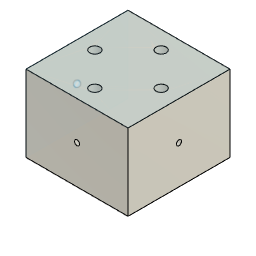
Suètone-drawing-object-02 (Autodesk Fusion 360 design; units mm, degrees)
Autodesk Fusion 360 part; units mm, degrees
sketch "Esquisse1" plane through (0, 0, 0) normal (0, 0, 1) x (1, 0, 0)
  line L0 (40, 40) -> (-40, 40)
  line L1 (-40, 40) -> (-40, -40)
  line L2 (-40, -40) -> (40, -40)
  line L3 (40, -40) -> (40, 40)
  line L4 (40, 40) -> (-40, -40) construction
  line L5 (-40, 40) -> (40, -40) construction
  dimension "d1" = 80
  dimension "d2" = 80
  constraint horizontal L0
  constraint perpendicular L0 L1
  constraint parallel L0 L2
  constraint parallel L1 L3
  constraint coincident L4 origin
  constraint coincident L5 origin
  measures "d1" distance of L1.end L2.end
  measures "d2" distance of L0.end L1.end
extrude "Extrusion1" add sketch "Esquisse1" along normal blind 80 makes body 1
sketch "Esquisse2" plane through (0, 0, 80) normal (0, 0, 1) x (-1, 0, 0)
  line L0 (-40, 40) -> (-40, -40)
  line L1 (-40, -40) -> (40, -40)
  line L2 (40, -40) -> (40, 40)
  line L3 (40, 40) -> (-40, 40)
  circle A0 centre (0, -26) radius 4
  circle A1 centre (26, 0) radius 4
  circle A2 centre (0, 26) radius 4
  circle A3 centre (-26, 0) radius 4
  dimension "d7" = 8
  dimension "d9" = 360
  measures "d7" diameter of A0
extrude "Extrusion2" cut sketch "Esquisse2" against normal blind 115 contours A0 | A1 | A2 | A3 bodies 1
sketch "Esquisse3" plane through (0, -40, 0) normal (0, -1, 0) x (1, 0, 0)
  line L0 (-40, 0) -> (40, 0)
  line L1 (40, 0) -> (40, 80)
  line L2 (40, 80) -> (-40, 80)
  line L3 (-40, 80) -> (-40, 0)
  line L4 (-40, 20) -> (40, 20)
  line L5 (40, 0, -80) -> (40, 80, -80)
  line L6 (40, 20, 0) -> (40, 20, -80)
  line L7 (-40, 0, -80) -> (-40, 80, -80)
  line L8 (40, 20, -80) -> (-40, 20, -80)
  line L9 (-40, 20, -80) -> (-40, 20, 0)
  constraint coincident L3 L4.start
  constraint coincident L1 L4.end
  constraint perpendicular L1 L4
ref_plane "Plan de construction1" through (0, 40, 20) normal (0, -0.707107, 0.707107) x (-1, 0, 0)
ref_plane "Plan de construction2" through (-40, 0, 20) normal (0.707107, 0, 0.707107) x (0, -1, 0)
ref_plane "Plan de construction3" through (0, -40, 20) normal (0, 0.707107, 0.707107) x (1, 0, 0)
ref_plane "Plan de construction4" through (40, 0, 20) normal (-0.707107, 0, 0.707107) x (0, 1, 0)
split "Scinder1" by plane through (40, 0, 20) normal (-0.707107, 0, 0.707107) bodies 1 makes body 2 at (-40, 13.3333, 26.6667)
split "Scinder2" by plane through (0, -40, 20) normal (0, 0.707107, 0.707107) bodies 2 makes body 3 at (-40, 20, 26.6667)
split "Scinder3" by plane through (-40, 0, 20) normal (0.707107, 0, 0.707107) bodies 3 makes body 4 at (-23.2337, 23.3296, 80)
split "Scinder4" by plane through (0, 40, 20) normal (0, -0.707107, 0.707107) bodies 4 makes body 5 at (-23.2337, 23.3296, 80)
delete_body "RemoveBody1" bodies 4
delete_body "RemoveBody2" bodies 1
delete_body "RemoveBody3" bodies 2
delete_body "RemoveBody4" bodies 3
sketch "Esquisse4" plane through (0, 0, 80) normal (0, 0, 1) x (-1, 0, 0)
  circle A0 centre (0, -26) radius 4
  circle A1 centre (-26, 0) radius 4
  circle A2 centre (26, 0) radius 4
  circle A3 centre (0, 26) radius 4
  line L0 (-40, 40) -> (-40, -40)
  line L1 (-40, -40) -> (40, -40)
  line L2 (40, -40) -> (40, 40)
  line L3 (40, 40) -> (-40, 40)
sketch "Esquisse5" plane through (0, 0, 80) normal (0, 0, 1) x (-1, 0, 0)
sketch "Esquisse6" plane through (40, 0, 0) normal (1, 0, 0) x (0, 1, 0)
  line L0 (-40, 20) -> (40, 20)
  line L1 (40, 20) -> (40, 80)
  line L2 (40, 80) -> (-40, 80)
  line L3 (-40, 80) -> (-40, 20)
  circle A0 centre (0, 50) radius 2
  dimension "d17" = 4
  measures "d17" diameter of A0
extrude "Extrusion3" cut sketch "Esquisse6" against normal blind 15 contours A0 bodies 5
sketch "Esquisse7" plane through (0, -40, 0) normal (0, -1, 0) x (1, 0, 0)
  line L0 (-40, 20) -> (40, 20)
  line L1 (40, 20) -> (40, 80)
  line L2 (40, 80) -> (-40, 80)
  line L3 (-40, 80) -> (-40, 20)
  circle A0 centre (0, 50) radius 2
  dimension "d20" = 4
  measures "d20" diameter of A0
extrude "Extrusion4" cut sketch "Esquisse7" against normal blind 13 contours A0 bodies 5
sketch "Esquisse8" plane through (-40, 0, 0) normal (-1, 0, 0) x (0, -1, 0)
  line L0 (-40, 20) -> (40, 20)
  line L1 (40, 20) -> (40, 80)
  line L2 (40, 80) -> (-40, 80)
  line L3 (-40, 80) -> (-40, 20)
  circle A0 centre (0, 50) radius 2
  dimension "d23" = 4
  measures "d23" diameter of A0
extrude "Extrusion5" [suppressed]
sketch "Esquisse9" plane through (0, 40, 0) normal (0, 1, 0) x (-1, 0, 0)
  line L0 (-40, 20) -> (40, 20)
  line L1 (40, 20) -> (40, 80)
  line L2 (40, 80) -> (-40, 80)
  line L3 (-40, 80) -> (-40, 20)
  circle A0 centre (0, 50) radius 2
  dimension "d26" = 4
  measures "d26" diameter of A0
extrude "Extrusion6" [suppressed]
sketch "Esquisse10" plane through (0, 0, 0) normal (0, 0, -1) x (1, 0, 0)
  line L0 (-20, -20) -> (20, -20)
  line L1 (20, -20) -> (20, 20)
  line L2 (20, 20) -> (-20, 20)
  line L3 (-20, 20) -> (-20, -20)
  line L4 (17, 18) -> (-17, 18)
  line L5 (-17, 18) -> (-17, 16)
  line L6 (17, 16) -> (17, 18)
  line L7 (17, 18) -> (-17, 18)
  line L8 (-17, 18) -> (-17, -18)
  line L9 (-17, -18) -> (17, -18)
  line L10 (17, -18) -> (17, 18)
  line L11 (17, 18) -> (-17, -18) construction
  line L12 (-17, 18) -> (17, -18) construction
  constraint perpendicular L4 L5
  constraint parallel L5 L6
  constraint horizontal L7
  constraint perpendicular L7 L8
  constraint parallel L8 L10
  constraint coincident L11 origin
  constraint coincident L12 origin
extrude "Extrusion7" [suppressed]
sketch "Esquisse11" plane through (0, 0, 80) normal (0, 0, 1) x (-1, 0, 0)
